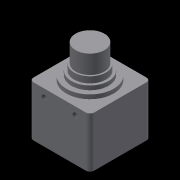
# Autodesk Inventor part: 3d_JacintoDevKit_Addon - Camera
Saved by Autodesk Inventor 2018.3 (Build 223284000, 284)
## iProperties
Created: 2026-02-24
Part Number: 3d_JacintoDevKit_Addon - Camera
Material: Genérico
Document SubType Name: Modeling
Designer: aca6
Density: 1 g/cm^3
Appearance: Valor por defecto
Author: aca6
Autodesk Inventor part; units mm, degrees
ref_plane "YZ Plane" through (0, 0, 0) normal (1, 0, 0) x (0, 1, 0)
ref_plane "XZ Plane" through (0, 0, 0) normal (0, 1, 0) x (-1, 0, 0)
ref_plane "XY Plane" through (0, 0, 0) normal (0, 0, 1) x (1, 0, 0)
sketch "Sketch1" plane through (0, 0, 0) normal (0, 0, 1) x (1, 0, 0)
  line L0 (-14.75, 14.75) -> (14.75, 14.75)
  line L1 (14.75, 14.75) -> (14.75, -14.75)
  line L2 (14.75, -14.75) -> (-14.75, -14.75)
  line L3 (-14.75, -14.75) -> (-14.75, 14.75)
  line L4 (0, 0) -> (0, 4.6825) construction
  line L5 (0, 0) -> (4.0135, 0) construction
  dimension "d0" = 29.5
  dimension "d1" = 29.5
  constraints: 12 end point, 3 horizontal, 2 parallel, 2 vertical, 1 perpendicular, 4 other
  measures "d0" distance of L0.start L0.end
  measures "d1" distance of L0.end L1.end
extrude "Extrusion1" add sketch "Sketch1" along normal blind 24.5
sketch "Sketch2" plane through (0, 0, 24.5) normal (0, 0, 1) x (1, 0, 0)
  circle A0 centre (0, 0) radius 11.5
  dimension "d4" = 23
  constraints: 1 centre point, 1 coincident
  measures "d4" diameter of A0
extrude "Extrusion2" add sketch "Sketch2" along normal blind 2
sketch "Sketch3" plane through (0, 0, 26.5) normal (0, 0, 1) x (1, 0, 0)
  circle A0 centre (0, 0) radius 9
  dimension "d7" = 18
  constraints: 1 centre point, 1 coincident
  measures "d7" diameter of A0
extrude "Extrusion3" add sketch "Sketch3" along normal blind 2
sketch "Sketch4" plane through (0, 0, 28.5) normal (0, 0, 1) x (1, 0, 0)
  circle A0 centre (0, 0) radius 7.75
  dimension "d10" = 15.5
  constraints: 1 centre point, 1 coincident
  measures "d10" diameter of A0
extrude "Extrusion4" add sketch "Sketch4" along normal blind 3
sketch "Sketch5" plane through (0, 0, 31.5) normal (0, 0, 1) x (1, 0, 0)
  circle A0 centre (0, 0) radius 7
  dimension "d13" = 14
  constraints: 1 centre point, 1 coincident
  measures "d13" diameter of A0
extrude "Extrusion5" add sketch "Sketch5" along normal blind 9
sketch "Sketch6" plane through (-14.75, 14.75, 0) normal (0, 1, 0) x (1, 0, 0)
  line L0 (29.5, -24.5) -> (0, -24.5) projected
  line L1 (0, 0) -> (0, -24.5) projected
  point P0 (14.75, 0)
  point P1 (7.25, -20.7)
  point P2 (22.25, -20.7)
  dimension "d16" = 15
  dimension "d17" = 3.8
  dimension "d18" = 7.25
  constraints: 1 horizontal alignment
  measures "d16" distance of point (22.25, -20.7) point (7.25, -20.7)
  measures "d17" distance from line of L0 point (7.25, -20.7)
  measures "d18" distance from line of L1 point (7.25, -20.7)
hole "Hole1" at (-7.5, 14.75, 20.7) at (7.5, 14.75, 20.7) direction (0, -1, 0) diameter 2.459 depth 3 tip angle 118 thread size "M3x0.5" class "6H" standard "ISO Metric profile"
fillet "Fillet1" radius 2 4 edges at (14.75, 14.75, 12.25) (-14.75, 14.75, 12.25) (-14.75, -14.75, 12.25) (14.75, -14.75, 12.25)
sketch "Sketch7" plane through (-12.75, -14.75, 0) normal (0, -1, 0) x (1, 0, 0)
  line L0 (0, 24.5) -> (25.5, 24.5) projected
  line L1 (-2, 24.5) -> (-2, 0) projected
  point P0 (12.75, 0)
  point P1 (5.25, 20.7)
  point P2 (20.25, 20.7)
  dimension "d27" = 15
  dimension "d28" = 3.8
  dimension "d29" = 7.25
  constraints: 1 horizontal alignment
  measures "d27" distance of point (20.25, 20.7) point (5.25, 20.7)
  measures "d28" distance from line of L0 point (20.25, 20.7)
  measures "d29" distance from line of L1 point (5.25, 20.7)
hole "Hole2" at (-7.5, -14.75, 20.7) at (7.5, -14.75, 20.7) direction (0, 1, 0) diameter 2.459 depth 3 tip angle 118 thread size "M3x0.5" class "6H" standard "ISO Metric profile"
sketch "Sketch8" plane through (0, 0, 0) normal (0, 0, -1) x (-1, 0, 0)
  line L0 (5.0435, 9.3) -> (-5.0435, 9.3) construction
  line L1 (3.15, 10.55) -> (-3.15, 10.55)
  line L2 (-3.15, 8.05) -> (3.15, 8.05)
  line L3 (0, 0) -> (-20.3594, 0) construction
  line L4 (0, 0) -> (0, -6.0077) construction
  line L5 (4.15, 9.05) -> (4.15, 9.55)
  line L6 (-4.15, 9.05) -> (-4.15, 9.55)
  arc A0 (3.15, 8.05) -> (4.15, 9.05) centre (3.15, 9.05) ccw
  arc A1 (4.15, 9.55) -> (3.15, 10.55) centre (3.15, 9.55) ccw
  arc A2 (-3.15, 10.55) -> (-4.15, 9.55) centre (-3.15, 9.55) ccw
  arc A3 (-4.15, 9.05) -> (-3.15, 8.05) centre (-3.15, 9.05) ccw
  point P0 (-4.15, 8.05)
  point P1 (4.15, 8.05)
  point P2 (0, 9.3)
  point P3 (-4.15, 10.55)
  dimension "d37" = 9.3
  dimension "d38" = 8.3
  dimension "d39" = 2.5
  dimension "d41" = 1
  constraints: 16 end point, 8 point on circle, 8 tangent, 6 point on line, 4 centre point, 3 equal radius, 3 horizontal, 3 vertical, 1 midpoint, 1 parallel, 1 perpendicular, 1 vertical alignment, 4 other
  measures "d37" distance between parallel lines of L3 L0
  measures "d38" distance of point (-4.15, 8.05) point (4.15, 8.05)
  measures "d39" distance of point (-4.15, 8.05) point (-4.15, 10.55)
  measures "d41" radius of A0
extrude "Extrusion6" cut sketch "Sketch8" against normal blind 6.5
body "Solid1"
